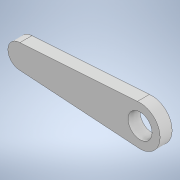
# Autodesk Inventor part: tail_end
Saved by Autodesk Inventor 2020.3 (Build 243373000, 373)
## iProperties
Created: 2020-08-15
Part Number: tail_end
Material: Generic
Document SubType Name: Modeling
Designer: aditk
Density: 1 g/cm^3
Appearance: Default
Author: aditk
Autodesk Inventor part; units mm, degrees
ref_plane "YZ Plane" through (0, 0, 0) normal (1, 0, 0) x (0, 1, 0)
ref_plane "XZ Plane" through (0, 0, 0) normal (0, 1, 0) x (-1, 0, 0)
ref_plane "XY Plane" through (0, 0, 0) normal (0, 0, 1) x (1, 0, 0)
sketch "Sketch1" plane through (0, 0, 0) normal (0, 0, 1) x (1, 0, 0)
  circle A0 centre (0, 0) radius 3
  circle A1 centre (0, 0) radius 5
  circle A2 centre (-30, 0) radius 3
  line L0 (-30, 3) -> (0, 5)
  line L1 (-30, -3) -> (0, -5)
  point P0 (-0.6637, -4.9558)
  point P1 (-0.6637, 4.9558)
  dimension "d0" = 6
  dimension "d1" = 10
  dimension "d2" = 6
  constraints: 4 end point, 4 point on circle, 3 centre point, 2 coincident
  measures "d0" diameter of A0
  measures "d1" diameter of A1
  measures "d2" diameter of A2
extrude "Extrusion1" add sketch "Sketch1" along normal blind 3
move faces "Move1" translate (0, 0, -15.25) faces at (-31.1759, 2.7599, 2)
body "Solid1"
